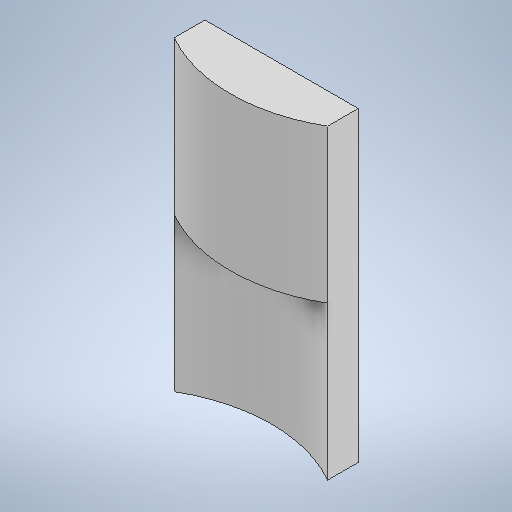
# Autodesk Inventor part: flat_surface_1
Saved by Autodesk Inventor 2025.1 (Build 291241000, 241)
## iProperties
Created: 2025-06-15
Part Number: flat_surface_1
Material: 일반
Document SubType Name: Modeling
Designer: USER
Density: 1 g/cm^3
Appearance: 기본값
Author: USER
Autodesk Inventor part; units mm, degrees
ref_plane "YZ Plane" through (0, 0, 0) normal (1, 0, 0) x (0, 1, 0)
ref_plane "XZ Plane" through (0, 0, 0) normal (0, 1, 0) x (-1, 0, 0)
ref_plane "XY Plane" through (0, 0, 0) normal (0, 0, 1) x (1, 0, 0)
sketch "스케치1" plane through (0, 0, 0) normal (0, 0, 1) x (1, 0, 0)
  line L0 (-0.15, 0) -> (0.9, 0) construction
  line L1 (0, -0.7) -> (0, 0.7) construction
  line L2 (0.25, -0.5) -> (0.75, -0.5)
  line L3 (0.75, -0.5) -> (0.75, 0.5)
  line L4 (0.75, 0.5) -> (0.25, 0.5)
  line L5 (0.25, 0.5) -> (0.25, -0.5)
  point P0 (0, 0)
  point P1 (0.5, -0.5)
  dimension "d7" = 0.5
  dimension "d8" = 1
  dimension "d9" = 0.25
  constraints: 8 end point, 2 parallel, 1 horizontal, 1 midpoint, 1 perpendicular, 1 other
  measures "d7" distance between parallel lines of L5 L3
  measures "d8" distance between parallel lines of L2 L4
  measures "d9" distance between parallel lines of L1 L5
extrude "돌출1" add sketch "스케치1" along normal blind 0.1
sketch "스케치3" plane through (0.25, 0.5, 0) normal (0, 1, 0) x (1, 0, 0)
  line L0 (-0.25, 0.6093) -> (-0.25, -0.2964) construction
  line L1 (-0.4, 0) -> (0.65, 0) construction
  line L2 (0.5, 0) -> (0, 0) projected
  line L3 (0, 0) -> (0, -0.1) projected
  line L4 (0.5, -0.1) -> (0, -0.1) projected
  line L5 (0.5, 0) -> (0.5, -0.1) projected
  arc A0 (0, -0.1) -> (0.5, -0.1) centre (0.25, 0.333) ccw
  line L6 (0.25, -0.1) -> (0.25, 0.4799) construction
  point P0 (-0.25, 0)
  dimension "d10" = 0.5
  constraints: 2 end point, 2 point on circle, 1 centre point, 1 midpoint, 1 point on line, 1 vertical
  measures "d10" radius of A0
extrude "돌출3" add sketch "스케치3" against normal blind 0.5 contours A0 L4
sketch "스케치4" plane through (0.25, -0.5, 0) normal (0, -1, 0) x (1, 0, 0)
  line L0 (0, 0) -> (0.5, 0) projected
  line L1 (0.5, 0) -> (0.5, 0.1) projected
  line L2 (0, 0.1) -> (0.5, 0.1) projected
  line L3 (0, 0) -> (0, 0.1) projected
  arc A0 (0, 0.1) -> (0.5, 0.1) centre (0.25, 0.533) ccw
  point P0 (-0.25, 0)
  dimension "d15" = 0.5
  constraints: 2 point on circle, 1 centre point
  measures "d15" radius of A0
extrude "돌출4" cut sketch "스케치4" against normal blind 0.5 contours L2 A0
